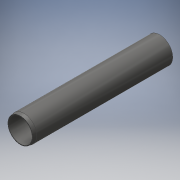
# Autodesk Inventor part: Cup_Dispenser_Pipe
Saved by Autodesk Inventor 2016 (Build 200138000, 138)
## iProperties
Created: 2015-07-03
Part Number: Cup_Dispenser_Pipe
Material: Generic
Document SubType Name: Modeling
Designer: bastli
Density: 1 g/cm^3
Appearance: Rubber - Black - Version 1.1
Author: bastli
Autodesk Inventor part; units mm, degrees
ref_plane "YZ Plane" through (0, 0, 0) normal (1, 0, 0) x (0, 1, 0)
ref_plane "XZ Plane" through (0, 0, 0) normal (0, 1, 0) x (-1, 0, 0)
ref_plane "XY Plane" through (0, 0, 0) normal (0, 0, 1) x (1, 0, 0)
sketch "Sketch1" plane through (0, 0, 0) normal (0, 1, 0) x (-1, 0, 0)
  circle A0 centre (0, 0) radius 37.5
  circle A1 centre (0, 0) radius 34
  dimension "d0" = 75
  dimension "d1" = 3.5
  constraints: 2 centre point, 1 coincident
  measures "d0" diameter of A0
  measures "d1" radial gap between concentric circles of A0 A1
extrude "Extrusion1" add sketch "Sketch1" along normal blind 400
sketch "Sketch2" plane through (0, 400, 0) normal (0, 1, 0) x (1, 0, 0)
  point P0 (0, 0)
chamfer "Chamfer2" distance 1.75 distance2 10 1 edges at (37.5, 0, 0) measured on face at (0, 0, 35.0014)
body "Solid1"
